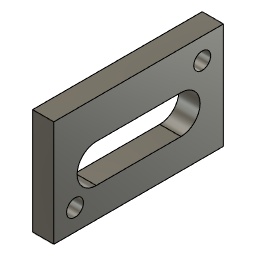
Регулировка под валлы v2 (Autodesk Fusion 360 design; units mm, degrees)
Autodesk Fusion 360 part; units mm, degrees
sketch "Sketch1" plane through (0, 0, 0) normal (1, 0, 0) x (0, 0, -1)
  line L0 (0, 0) -> (40, 0)
  line L1 (40, 0) -> (40, 25)
  line L2 (40, 25) -> (0, 25)
  line L3 (0, 25) -> (0, 0)
  circle A0 centre (35, 20) radius 2
  circle A1 centre (5, 5) radius 2
  line L4 (10, 16) -> (30, 16)
  arc A2 (30, 7) -> (30, 16) centre (30, 11.5) ccw
  line L5 (30, 7) -> (10, 7)
  arc A3 (10, 16) -> (10, 7) centre (10, 11.5) ccw
  dimension "d1" = 40
  dimension "d2" = 25
  dimension "d3" = 4
  dimension "d4" = 4
  dimension "d5" = 5
  dimension "d7" = 35
  dimension "d8" = 5
  dimension "d9" = 35
  dimension "d10" = 9
  dimension "d11" = 20
  dimension "d12" = 7
  dimension "d14" = 10
  constraint horizontal L0
  constraint vertical L1
  constraint horizontal L2
  constraint vertical L3
  constraint coincident L0.start L3.end
  constraint parallel L2 L4
  constraint tangent L4 A2
  constraint tangent A2 L5
  constraint parallel L4 L5
  constraint tangent L5 A3
  constraint tangent L4 A3
  measures "d1" distance of L0.start L0.end
  measures "d2" distance of L0.start L2.end
  measures "d3" diameter of A0
  measures "d4" diameter of A1
  measures "d5" distance of L0 A1.centre
  measures "d7" distance of L1 A1.centre
  measures "d8" distance of L2 A0.centre
  measures "d9" distance of L3 A0.centre
  measures "d10" distance of L2 L4
  measures "d11" distance of A2.start L5.end
  measures "d12" distance of L0 L5
  measures "d14" distance of L1 A2.centre
extrude "Extrude1" add sketch "Sketch1" along normal blind 5
